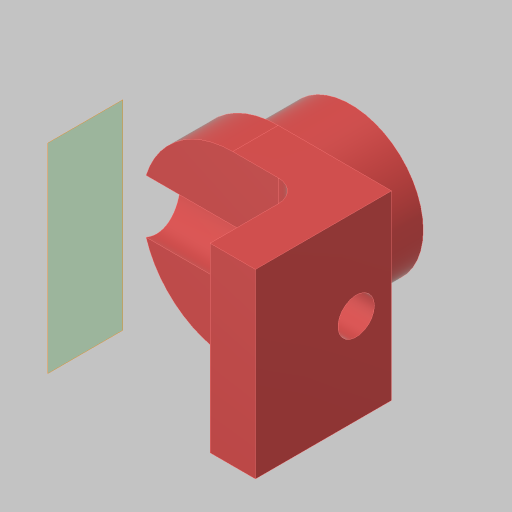
# Autodesk Inventor part: constant force Spring Holder 2
Saved by Autodesk Inventor 2023.5 (Build 275446000, 446)
## iProperties
Created: 2025-01-21
Part Number: constant force Spring Holder 2
Material: ABS Plastic
Document SubType Name: Modeling
Designer: slick
Density: 1.06 g/cm^3
Appearance: Smooth - Red
Author: slick
Autodesk Inventor part; units mm, degrees
ref_plane "YZ Plane" through (0, 0, 0) normal (1, 0, 0) x (0, 1, 0)
ref_plane "XZ Plane" through (0, 0, 0) normal (0, 1, 0) x (-1, 0, 0)
ref_plane "XY Plane" through (0, 0, 0) normal (0, 0, 1) x (1, 0, 0)
sketch "Sketch1" plane through (0, 0, 0) normal (0, 0, 1) x (1, 0, 0)
  circle A0 centre (0, 0) radius 10.16
  circle A1 centre (0, 0) radius 8.7376
  dimension "d0" = 20.32
  dimension "d6" = 17.4752
  constraints: 2 centre point, 2 coincident
  measures "d0" diameter of A0
  measures "d6" diameter of A1
extrude "Extrusion1" add sketch "Sketch1" along normal blind 10.16 contours A0 | A1
sketch "Sketch2" plane through (0, 0, 10.16) normal (0, 0, 1) x (1, 0, 0)
  circle A0 centre (0, 0) radius 10.16 projected
  circle A1 centre (0, 0) radius 12.7 construction
  line L0 (0, 12.7) -> (15.875, 12.7)
  line L1 (15.875, 12.7) -> (15.875, -12.7)
  line L2 (15.875, -12.7) -> (0, -12.7)
  arc A2 (0, 12.7) -> (0, -12.7) centre (0, 0) ccw
  point P0 (15.875, 0)
  dimension "d3" = 2.54
  dimension "d14" = 15.875
  dimension "d35" = 25.4
  constraints: 6 end point, 4 point on circle, 2 centre point, 2 horizontal, 1 coincident, 1 horizontal alignment, 1 midpoint, 1 perpendicular, 1 tangent
  measures "d3" radial gap between concentric circles of A0 A1
  measures "d14" distance of L0.start L0.end
  measures "d35" distance of L0.end L1.end
extrude "Extrusion2" add sketch "Sketch2" along normal blind 6.35 contours A0 | L0 L1 L2 A2
sketch "Sketch4" plane through (0, 0, 16.51) normal (0, 0, 1) x (1, 0, 0)
  arc A0 (0, 12.7) -> (0, -12.7) centre (0, 0) ccw projected
  constraints: 1 coincident
hole "Hole2" at (0, 0, 16.51) direction (0, 0, -1) diameter 6.5278 end through all clearance for "Flat Head Machine Screw (82)" size "1/4" standard "Ansi Unified Screw Threads"
sketch "Sketch5" plane through (0, 0, 16.51) normal (0, 0, 1) x (1, 0, 0)
  line L0 (15.875, 12.7) -> (0, 12.7) projected
  line L1 (0, -12.7) -> (15.875, -12.7) projected
  line L2 (15.875, 12.7) -> (9.525, 12.7)
  line L3 (9.525, 12.7) -> (9.525, -12.7)
  line L4 (9.525, -12.7) -> (15.875, -12.7)
  line L5 (15.875, -12.7) -> (15.875, 12.7)
  point P0 (0, 0)
  dimension "d22" = 6.35
  constraints: 8 end point, 2 parallel, 1 horizontal, 1 perpendicular, 1 point on line
  measures "d22" distance between parallel lines of L5 L3
extrude "Extrusion3" add sketch "Sketch5" along normal blind 12.7
fillet "Fillet1" radius 3.175 1 edges at (9.525, 0, 16.51)
sketch "Sketch6" plane through (15.875, -12.7, 10.16) normal (1, 0, 0) x (0, 0, -1)
  line L0 (-12.7, 19.05) -> (-12.7, 6.35) construction
  line L1 (-19.05, 0) -> (-19.05, 25.4) construction
  line L2 (0, 25.4) -> (-19.05, 25.4) construction
  point P0 (10.16, 12.7)
  point P1 (-12.7, 12.7)
  point P2 (-19.05, 12.7)
  point P3 (-9.525, 25.4)
  point P4 (-4.953, 12.7)
  dimension "d26" = 12.7
  dimension "d34" = 6.35
  dimension "d36" = 14.097
  constraints: 3 midpoint, 2 end point, 2 horizontal alignment, 1 vertical, 1 vertical alignment
  measures "d26" distance of L0.start L0.end
  measures "d34" distance between parallel lines of L1 L0
  measures "d36" distance from line of L1 point (-4.953, 12.7)
hole "Hole3" at (15.875, 0, 15.113) direction (-1, 0, 0) diameter 5.1054 end through all clearance for "Flat Head Machine Screw (82)" size "#10" standard "Ansi Unified Screw Threads"
ref_plane "Work Plane1" through (-12.7, -12.7, 29.21) normal (-1, 0, 0) x (0, 0, 1)
sketch "Sketch7" plane through (-12.7, -12.7, 29.21) normal (-1, 0, 0) x (0, 0, 1)
  line L0 (-19.05, 12.7) -> (-16.6497, 12.7) construction
  line L1 (-19.05, 12.7) -> (-16.6497, 12.7) construction
  circle A0 centre (-14.097, 12.7) radius 2.5527 construction
  circle A1 centre (-14.097, 12.7) radius 4.0005
  point P0 (-29.21, 12.7)
  dimension "d38" = 8.001
  constraints: 1 centre point, 1 coincident, 1 other
  measures "d38" diameter of A1
extrude "Extrusion4" cut sketch "Sketch7" against normal blind 20.32
body "Solid1"
